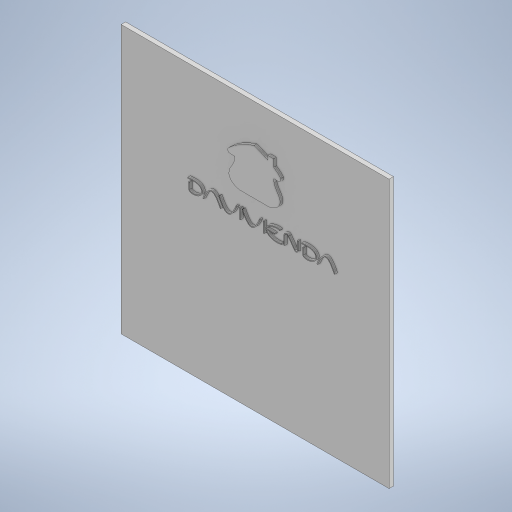
# Autodesk Inventor part: Davivienda
Saved by Autodesk Inventor 2023 (Build 270158000, 158)
## iProperties
Created: 2024-11-21
Part Number: Davivienda
Material: Generic
Document SubType Name: Modeling
Designer: Zenbook
Density: 1 g/cm^3
Appearance: Default
Author: Zenbook
Autodesk Inventor part; units mm, degrees
ref_plane "YZ Plane" through (0, 0, 0) normal (1, 0, 0) x (0, 1, 0)
ref_plane "XZ Plane" through (0, 0, 0) normal (0, 1, 0) x (-1, 0, 0)
ref_plane "XY Plane" through (0, 0, 0) normal (0, 0, 1) x (1, 0, 0)
sketch "Sketch2" plane through (0, 0, 0) normal (0, 0, 1) x (1, 0, 0)
  line L0 (0, 0) -> (300, 0)
  line L1 (300, 0) -> (300, 300)
  line L2 (300, 300) -> (0, 300)
  line L3 (0, 300) -> (0, 0)
  dimension "d0" = 300
  dimension "d1" = 300
  constraints: 8 end point, 2 parallel, 1 horizontal, 1 perpendicular
  measures "d0" distance of L2.end L1.end
  measures "d1" distance of L1.end L0.end
extrude "Extrusion1" add sketch "Sketch2" along normal blind 5
sketch "Sketch4" plane through (0, 0, 5) normal (0, 0, 1) x (1, 0, 0)
  line L0 (79.5564, 188.2855) -> (79.5564, 181.2855)
  line L1 (79.5564, 181.2855) -> (79.5564, 178.6599) construction
  line L2 (79.5564, 178.6599) -> (94.7024, 178.6599) construction
  line L3 (94.7024, 178.6599) -> (96.5971, 188.6652) construction
  line L4 (96.5971, 188.6652) -> (88.3362, 192.4913) construction
  line L5 (88.3362, 192.4913) -> (77.7258, 191.1271) construction
  spline S0 degree 4 poles (79.5564, 181.2855) (79.5564, 178.6599) (94.7024, 178.6599) (96.5971, 188.6652) (88.3362, 192.4913) (77.7258, 191.1271) knots 1 1 1 1 1 2 3 3 3 3 3
  line L6 (95.2867, 179.9727) -> (97.8294, 186.2811) construction
  line L7 (97.8294, 186.2811) -> (104.3309, 202.3418) construction
  line L8 (104.3309, 202.3418) -> (110.5428, 186.2811) construction
  line L9 (110.5428, 186.2811) -> (113.8579, 179.9727) construction
  spline S1 degree 4 poles (95.2867, 179.9727) (97.8294, 186.2811) (104.3309, 202.3418) (110.5428, 186.2811) (113.8579, 179.9727) knots 1 1 1 1 1 2 2 2 2 2
  line L10 (131.5825, 191.7075) -> (129.0398, 185.3991) construction
  line L11 (129.0398, 185.3991) -> (122.5383, 169.3383) construction
  line L12 (122.5383, 169.3383) -> (116.3264, 185.3991) construction
  line L13 (116.3264, 185.3991) -> (113.0113, 191.7075) construction
  spline S2 degree 4 poles (131.5825, 191.7075) (129.0398, 185.3991) (122.5383, 169.3383) (116.3264, 185.3991) (113.0113, 191.7075) knots 1 1 1 1 1 2 2 2 2 2
  spline S3 degree 4 poles (157.762, 191.8087) (155.2194, 185.5002) (148.7178, 169.4395) (142.5059, 185.5002) (139.1908, 191.8087) knots 1 1 1 1 1 2 2 2 2 2
  line L14 (157.762, 191.8087) -> (155.2194, 185.5002) construction
  line L15 (155.2194, 185.5002) -> (148.7178, 169.4395) construction
  line L16 (148.7178, 169.4395) -> (142.5059, 185.5002) construction
  line L17 (142.5059, 185.5002) -> (139.1908, 191.8087) construction
  line L18 (135.5149, 191.7075) -> (135.5149, 180.2075)
  line L19 (162.0018, 191.8085) -> (162.0018, 180.3085)
  line L20 (180.6346, 191.8085) -> (171.5415, 194.3115) construction
  line L21 (171.5415, 194.3115) -> (152.9228, 186.4259) construction
  line L22 (152.9228, 186.4259) -> (171.5415, 176.543) construction
  line L23 (171.5415, 176.543) -> (182.4118, 180.3085) construction
  spline S4 degree 4 poles (180.6346, 191.8085) (171.5415, 194.3115) (152.9228, 186.4259) (171.5415, 176.543) (182.4118, 180.3085) knots 1 1 1 1 1 2 2 2 2 2
  line L24 (165.8328, 186.4259) -> (174.8813, 186.4259)
  line L25 (186.057, 180.0241) -> (186.057, 189.935)
  line L26 (189.8603, 191.1584) -> (197.0204, 180.9967)
  line L27 (201.0713, 182.1524) -> (201.0713, 191.8085)
  arc A0 (189.8811, 191.1289) -> (186.057, 189.935) centre (188.1554, 189.935) ccw
  arc A1 (197.0204, 180.9967) -> (201.0713, 182.1524) centre (198.8441, 182.2817) ccw
  line L28 (207.2296, 188.507) -> (207.2296, 181.507)
  line L29 (207.2296, 181.507) -> (207.2296, 178.8814) construction
  line L30 (207.2296, 178.8814) -> (222.3756, 178.8814) construction
  line L31 (222.3756, 178.8814) -> (224.2703, 188.8868) construction
  line L32 (224.2703, 188.8868) -> (216.0093, 192.7129) construction
  line L33 (216.0093, 192.7129) -> (205.3989, 191.3487) construction
  spline S5 degree 4 poles (207.2296, 181.507) (207.2296, 178.8814) (222.3756, 178.8814) (224.2703, 188.8868) (216.0093, 192.7129) (205.3989, 191.3487) knots 1 1 1 1 1 2 3 3 3 3 3
  line L34 (222.9422, 180.0767) -> (225.4849, 186.3851) construction
  line L35 (225.4849, 186.3851) -> (231.9865, 202.4459) construction
  line L36 (231.9865, 202.4459) -> (238.1983, 186.3851) construction
  line L37 (238.1983, 186.3851) -> (241.5135, 180.0767) construction
  spline S6 degree 4 poles (222.9422, 180.0767) (225.4849, 186.3851) (231.9865, 202.4459) (238.1983, 186.3851) (241.5135, 180.0767) knots 1 1 1 1 1 2 2 2 2 2
  line L38 (135.9918, 208.9074) -> (168.4766, 208.9074)
  line L39 (167.2414, 253.646) -> (167.2414, 258.1826)
  line L40 (167.2414, 258.1826) -> (173.7908, 258.1826)
  line L41 (173.7908, 258.1826) -> (173.7908, 249.9244)
  line L42 (135.9918, 208.9074) -> (128.025, 210.0808) construction
  line L43 (128.025, 210.0808) -> (119.7557, 218.4745) construction
  line L44 (119.7557, 218.4745) -> (124.3195, 226.1379) construction
  line L45 (124.3195, 226.1379) -> (130.2483, 231.5726) construction
  line L46 (130.2483, 231.5726) -> (130.2483, 238.8487) construction
  spline S7 degree 4 poles (135.9918, 208.9074) (128.025, 210.0808) (119.7557, 218.4745) (124.3195, 226.1379) (130.2483, 231.5726) (130.2483, 238.8487) knots 1 1 1 1 1 2 3 3 3 3 3
  line L47 (168.4766, 208.9074) -> (175.8602, 210.0808) construction
  line L48 (175.8602, 210.0808) -> (186.1394, 218.4745) construction
  line L49 (186.1394, 218.4745) -> (179.0921, 227.5218) construction
  line L50 (179.0921, 227.5218) -> (173.9355, 231.5726) construction
  line L51 (173.9355, 231.5726) -> (173.9355, 238.8487) construction
  spline S8 degree 4 poles (168.4766, 208.9074) (175.8602, 210.0808) (186.1394, 218.4745) (179.0921, 227.5218) (173.9355, 231.5726) (173.9355, 238.8487) knots 1 1 1 1 1 2 3 3 3 3 3
  line L52 (123.2696, 243.6155) -> (134.5896, 254.6512) construction
  line L53 (134.5896, 254.6512) -> (152.0248, 260.2524) construction
  spline S9 degree 2 poles (123.2696, 243.6155) (134.5896, 254.6512) (152.0248, 260.2524) knots 1 1 1 2 2 2
  line L54 (152.0248, 260.2524) -> (160.8389, 256.9124) construction
  line L55 (179.2014, 246.4492) -> (181.8101, 243.0596) construction
  arc A2 (123.2696, 243.6155) -> (124.9575, 238.8487) centre (124.9575, 241.5309) ccw
  arc A3 (179.0921, 238.8487) -> (181.8101, 243.0596) centre (179.0921, 241.8313) ccw
  line L56 (124.9575, 238.8487) -> (130.2483, 238.8487)
  line L57 (173.9355, 238.8487) -> (179.0921, 238.8487)
  spline S10 degree 2 poles (152.0248, 260.2524) (160.8389, 256.9124) (167.2414, 253.646) knots 0 0 0 1 1 1
  spline S11 degree 2 poles (173.7908, 249.9244) (179.2014, 246.4492) (181.8101, 243.0596) knots 0 0 0 1 1 1
  line L58 (160.8389, 256.9124) -> (167.2414, 253.646) construction
  line L59 (173.7908, 249.9244) -> (179.2014, 246.4492) construction
  point P0 (0, 0)
  point P1 (175.3935, 251.397)
  dimension "d11" = 7
  dimension "d28" = 11.5
  dimension "d29" = 11.5
  dimension "d42" = 7
  constraints: 28 end point, 9 point on circle, 7 vertical, 6 tangent, 4 centre point, 4 horizontal, 4 perpendicular, 1 point on line, 37 other
  measures "d11" distance of L0.start L0.end
  measures "d28" distance of L18.start L18.end
  measures "d29" distance of L19.start L19.end
  measures "d42" distance of L28.start L29.start
extrude "Extrusion2" add sketch "Sketch4" along normal blind 3
sketch "Sketch6" plane through (0, 0, 5) normal (0, 0, 1) x (1, 0, 0)
  line L0 (79.5564, 188.2855) -> (79.5564, 181.2855)
  line L1 (79.5564, 181.2855) -> (79.5564, 178.6599) construction
  line L2 (79.5564, 178.6599) -> (94.7024, 178.6599) construction
  line L3 (94.7024, 178.6599) -> (96.5971, 188.6652) construction
  line L4 (96.5971, 188.6652) -> (88.3362, 192.4913) construction
  line L5 (88.3362, 192.4913) -> (77.7258, 191.1271) construction
  spline S0 degree 4 poles (79.5564, 181.2855) (79.5564, 178.6599) (94.7024, 178.6599) (96.5971, 188.6652) (88.3362, 192.4913) (77.7258, 191.1271) knots 1 1 1 1 1 2 3 3 3 3 3
  line L6 (95.2867, 179.9727) -> (97.8294, 186.2811) construction
  line L7 (97.8294, 186.2811) -> (104.3309, 202.3418) construction
  line L8 (104.3309, 202.3418) -> (110.5428, 186.2811) construction
  line L9 (110.5428, 186.2811) -> (113.8579, 179.9727) construction
  spline S1 degree 4 poles (95.2867, 179.9727) (97.8294, 186.2811) (104.3309, 202.3418) (110.5428, 186.2811) (113.8579, 179.9727) knots 1 1 1 1 1 2 2 2 2 2
  spline S2 degree 4 poles (131.5825, 191.7075) (129.0398, 185.3991) (122.5383, 169.3383) (116.3264, 185.3991) (113.0113, 191.7075) knots 1 1 1 1 1 2 2 2 2 2
  line L10 (131.5825, 191.7075) -> (129.0398, 185.3991) construction
  line L11 (129.0398, 185.3991) -> (122.5383, 169.3383) construction
  line L12 (122.5383, 169.3383) -> (116.3264, 185.3991) construction
  line L13 (116.3264, 185.3991) -> (113.0113, 191.7075) construction
  spline S3 degree 4 poles (157.762, 191.8087) (155.2194, 185.5002) (148.7178, 169.4395) (142.5059, 185.5002) (139.1908, 191.8087) knots 1 1 1 1 1 2 2 2 2 2
  line L14 (157.762, 191.8087) -> (155.2194, 185.5002) construction
  line L15 (155.2194, 185.5002) -> (148.7178, 169.4395) construction
  line L16 (148.7178, 169.4395) -> (142.5059, 185.5002) construction
  line L17 (142.5059, 185.5002) -> (139.1908, 191.8087) construction
  line L18 (135.5149, 191.7075) -> (135.5149, 180.2075)
  line L19 (162.0018, 191.8085) -> (162.0018, 180.3085)
  line L20 (180.6346, 191.8085) -> (171.5415, 194.3115) construction
  line L21 (171.5415, 194.3115) -> (152.9228, 186.4259) construction
  line L22 (152.9228, 186.4259) -> (171.5415, 176.543) construction
  line L23 (171.5415, 176.543) -> (182.4118, 180.3085) construction
  spline S4 degree 4 poles (180.6346, 191.8085) (171.5415, 194.3115) (152.9228, 186.4259) (171.5415, 176.543) (182.4118, 180.3085) knots 1 1 1 1 1 2 2 2 2 2
  line L24 (165.8328, 186.4259) -> (174.8813, 186.4259)
  line L25 (186.057, 180.0241) -> (186.057, 189.935)
  line L26 (189.8603, 191.1584) -> (197.0204, 180.9967)
  line L27 (201.0713, 182.1524) -> (201.0713, 191.8085)
  arc A0 (189.8811, 191.1289) -> (186.057, 189.935) centre (188.1554, 189.935) ccw
  arc A1 (197.0204, 180.9967) -> (201.0713, 182.1524) centre (198.8441, 182.2817) ccw
  spline S5 degree 4 poles (207.2296, 181.507) (207.2296, 178.8814) (222.3756, 178.8814) (224.2703, 188.8868) (216.0093, 192.7129) (205.3989, 191.3487) knots 1 1 1 1 1 2 3 3 3 3 3
  line L28 (207.2296, 181.507) -> (207.2296, 178.8814) construction
  line L29 (207.2296, 178.8814) -> (222.3756, 178.8814) construction
  line L30 (222.3756, 178.8814) -> (224.2703, 188.8868) construction
  line L31 (224.2703, 188.8868) -> (216.0093, 192.7129) construction
  line L32 (216.0093, 192.7129) -> (205.3989, 191.3487) construction
  line L33 (207.2296, 188.507) -> (207.2296, 181.507)
  spline S6 degree 4 poles (222.9422, 180.0767) (225.4849, 186.3851) (231.9865, 202.4459) (238.1983, 186.3851) (241.5135, 180.0767) knots 1 1 1 1 1 2 2 2 2 2
  line L34 (222.9422, 180.0767) -> (225.4849, 186.3851) construction
  line L35 (225.4849, 186.3851) -> (231.9865, 202.4459) construction
  line L36 (231.9865, 202.4459) -> (238.1983, 186.3851) construction
  line L37 (238.1983, 186.3851) -> (241.5135, 180.0767) construction
  line L38 (78.5564, 181.2855) -> (78.5564, 188.2855)
  line L39 (136.5149, 191.7075) -> (136.5149, 180.2075)
  line L40 (163.0018, 191.8085) -> (163.0018, 180.3085)
  line L41 (165.8565, 185.4259) -> (174.8813, 185.4259)
  line L42 (185.057, 180.0241) -> (185.057, 189.935)
  arc A2 (190.7035, 191.6979) -> (185.057, 189.935) centre (188.1554, 189.935) ccw
  line L43 (190.6778, 191.7344) -> (197.8379, 181.5727)
  arc A3 (197.8379, 181.5727) -> (200.0713, 182.1857) centre (198.8441, 182.2817) ccw
  line L44 (200.0713, 182.1857) -> (200.0713, 191.8085)
  line L45 (206.2296, 181.507) -> (206.2296, 188.507)
  line L46 (79.5564, 188.2855) -> (78.5564, 188.2855)
  line L47 (77.7258, 191.1271) -> (77.5982, 192.1189)
  line L48 (95.2867, 179.9727) -> (94.3592, 180.3465)
  line L49 (113.8579, 179.9727) -> (114.7431, 180.4378)
  line L50 (112.1261, 191.2423) -> (113.0113, 191.7075)
  line L51 (132.51, 191.3337) -> (131.5825, 191.7075)
  line L52 (135.5149, 191.7075) -> (136.5149, 191.7075)
  line L53 (135.5149, 180.2075) -> (136.5149, 180.2075)
  line L54 (138.3056, 191.3435) -> (139.1908, 191.8087)
  line L55 (157.762, 191.8087) -> (158.6895, 191.4348)
  line L56 (162.0018, 191.8085) -> (163.0018, 191.8085)
  line L57 (162.0018, 180.3085) -> (163.0018, 180.3085)
  line L58 (182.7391, 179.3635) -> (182.4118, 180.3085)
  line L59 (174.8813, 185.4259) -> (174.8813, 186.4259)
  line L60 (185.057, 180.0241) -> (186.057, 180.0241)
  line L61 (200.0713, 191.8085) -> (201.0713, 191.8085)
  line L62 (205.3989, 191.3487) -> (205.2714, 192.3405)
  line L63 (206.2296, 188.507) -> (207.2296, 188.507)
  line L64 (222.0147, 180.4505) -> (222.9422, 180.0767)
  line L65 (241.5135, 180.0767) -> (242.3987, 180.5419)
  line L66 (180.6346, 191.8085) -> (180.9, 192.7726)
  spline S7 degree 5 poles (77.5982, 192.1189) (78.6162, 192.2498) (79.6368, 192.3603) (80.6599, 192.4464) (82.4837, 192.5473) (84.3098, 192.5266) (85.1087, 192.4899) (86.5329, 192.3645) (87.9377, 192.1029) (88.5503, 191.9568) (89.6455, 191.6249) (90.6851, 191.1491) (91.1369, 190.903) (91.9401, 190.3755) (92.6391, 189.7178) (92.9357, 189.3838) (93.4406, 188.6884) (93.8, 187.9087) (93.9352, 187.5178) (94.1241, 186.7215) (94.155, 185.9038) (94.1312, 185.4984) (94.0058, 184.6818) (93.7337, 183.9014) (93.5597, 183.5177) (93.1316, 182.7565) (92.5837, 182.0758) (92.2726, 181.7464) (91.5774, 181.1067) (90.8033, 180.5642) (90.3835, 180.3067) (89.4876, 179.8223) (88.5464, 179.433) (88.0508, 179.2556) (87.0359, 178.9432) (85.9973, 178.7219) (85.4688, 178.633) (84.4327, 178.5055) (83.3893, 178.4743) (82.8811, 178.4845) (81.9175, 178.556) (80.9731, 178.7614) (80.5348, 178.8931) (79.6638, 179.2662) (78.9659, 179.9065) (78.6841, 180.3256) (78.5566, 180.8089) (78.5564, 181.2855) knots 0 0 0 0 0 0 0.12687 0.12687 0.12687 0.225646 0.225646 0.225646 0.30335 0.30335 0.30335 0.36672 0.36672 0.36672 0.421609 0.421609 0.421609 0.472388 0.472388 0.472388 0.522285 0.522285 0.522285 0.5741 0.5741 0.5741 0.629898 0.629898 0.629898 0.690657 0.690657 0.690657 0.755632 0.755632 0.755632 0.821798 0.821798 0.821798 0.884532 0.884532 0.884532 0.940955 0.940955 0.940955 1 1 1 1 1 1
  spline S8 degree 5 poles (94.3592, 180.3465) (94.6691, 181.116) (94.9805, 181.8849) (95.3032, 182.6493) (96.0129, 184.2544) (96.7976, 185.8242) (97.2377, 186.6387) (98.1315, 188.1503) (99.1811, 189.559) (99.7178, 190.1922) (100.829, 191.292) (102.1665, 192.0911) (102.8464, 192.374) (104.2911, 192.6572) (105.7357, 192.373) (106.4176, 192.0904) (107.7678, 191.2937) (108.8988, 190.2004) (109.4502, 189.57) (110.5378, 188.1657) (111.4812, 186.6617) (111.9519, 185.8509) (112.8049, 184.2881) (113.6061, 182.6979) (113.9804, 181.9424) (114.3511, 181.1846) (114.7431, 180.4378) knots 0 0 0 0 0 0 0.124856 0.124856 0.124856 0.264073 0.264073 0.264073 0.388815 0.388815 0.388815 0.497298 0.497298 0.497298 0.606144 0.606144 0.606144 0.732055 0.732055 0.732055 0.87307 0.87307 0.87307 1 1 1 1 1 1
  spline S9 degree 5 poles (132.51, 191.3337) (132.2, 190.5642) (131.8887, 189.7952) (131.566, 189.0309) (130.8563, 187.4257) (130.0715, 185.8559) (129.6315, 185.0414) (128.7377, 183.5299) (127.6881, 182.1212) (127.1514, 181.488) (126.0402, 180.3882) (124.7026, 179.5891) (124.0227, 179.3061) (122.5781, 179.023) (121.1335, 179.3071) (120.4516, 179.5897) (119.1014, 180.3864) (117.9703, 181.4798) (117.4189, 182.1102) (116.3314, 183.5145) (115.388, 185.0184) (114.9173, 185.8293) (114.0642, 187.392) (113.2631, 188.9823) (112.8887, 189.7378) (112.518, 190.4956) (112.1261, 191.2423) knots 0 0 0 0 0 0 0.124856 0.124856 0.124856 0.264073 0.264073 0.264073 0.388815 0.388815 0.388815 0.497298 0.497298 0.497298 0.606144 0.606144 0.606144 0.732055 0.732055 0.732055 0.87307 0.87307 0.87307 1 1 1 1 1 1
  spline S10 degree 5 poles (158.6895, 191.4348) (158.3796, 190.6653) (158.0682, 189.8964) (157.7455, 189.1321) (157.0358, 187.5269) (156.2511, 185.9571) (155.811, 185.1426) (154.9172, 183.631) (153.8676, 182.2223) (153.3309, 181.5891) (152.2197, 180.4894) (150.8822, 179.6902) (150.2023, 179.4073) (148.7576, 179.1242) (147.3131, 179.4083) (146.6311, 179.6909) (145.2809, 180.4876) (144.1499, 181.5809) (143.5985, 182.2113) (142.5109, 183.6156) (141.5675, 185.1196) (141.0968, 185.9304) (140.2438, 187.4932) (139.4426, 189.0834) (139.0683, 189.8389) (138.6976, 190.5967) (138.3056, 191.3435) knots 0 0 0 0 0 0 0.124856 0.124856 0.124856 0.264073 0.264073 0.264073 0.388815 0.388815 0.388815 0.497298 0.497298 0.497298 0.606144 0.606144 0.606144 0.732055 0.732055 0.732055 0.87307 0.87307 0.87307 1 1 1 1 1 1
  spline S11 degree 5 poles (180.9, 192.7726) (179.961, 193.031) (178.9925, 193.1803) (178.0185, 193.2514) (176.0567, 193.2587) (174.1104, 193.0159) (173.1409, 192.8357) (171.3349, 192.3844) (169.6037, 191.6996) (168.8139, 191.3211) (167.4152, 190.5034) (166.2218, 189.4139) (165.7328, 188.8525) (164.9739, 187.6153) (164.7208, 186.1884) (164.7518, 185.476) (165.1202, 184.0479) (165.9664, 182.8345) (166.4989, 182.2761) (167.7984, 181.1743) (169.2947, 180.3514) (170.1475, 179.9675) (172.0371, 179.2718) (174.0038, 178.8379) (175.0707, 178.6746) (177.2645, 178.4828) (179.4643, 178.6019) (180.5798, 178.7493) (181.6801, 178.9966) (182.7391, 179.3635) knots 0 0 0 0 0 0 0.11949 0.11949 0.11949 0.240188 0.240188 0.240188 0.347394 0.347394 0.347394 0.437627 0.437627 0.437627 0.522195 0.522195 0.522195 0.615974 0.615974 0.615974 0.730426 0.730426 0.730426 0.862485 0.862485 0.862485 1 1 1 1 1 1
  spline S12 degree 5 poles (205.2714, 192.3405) (206.2894, 192.4714) (207.3099, 192.5819) (208.333, 192.668) (210.1569, 192.7689) (211.983, 192.7482) (212.7819, 192.7115) (214.206, 192.5861) (215.6109, 192.3244) (216.2234, 192.1784) (217.3186, 191.8464) (218.3583, 191.3707) (218.8101, 191.1245) (219.6132, 190.597) (220.3122, 189.9393) (220.6089, 189.6054) (221.1138, 188.91) (221.4732, 188.1302) (221.6084, 187.7394) (221.7973, 186.9431) (221.8282, 186.1254) (221.8043, 185.7199) (221.679, 184.9033) (221.4069, 184.123) (221.2328, 183.7393) (220.8047, 182.978) (220.2569, 182.2974) (219.9458, 181.968) (219.2505, 181.3283) (218.4765, 180.7858) (218.0566, 180.5283) (217.1608, 180.0439) (216.2195, 179.6546) (215.724, 179.4772) (214.709, 179.1648) (213.6704, 178.9435) (213.1419, 178.8546) (212.1058, 178.7271) (211.0625, 178.6959) (210.5542, 178.7061) (209.5906, 178.7776) (208.6462, 178.983) (208.2079, 179.1147) (207.337, 179.4878) (206.6391, 180.128) (206.3572, 180.5472) (206.2297, 181.0305) (206.2296, 181.507) knots 0 0 0 0 0 0 0.12687 0.12687 0.12687 0.225646 0.225646 0.225646 0.30335 0.30335 0.30335 0.36672 0.36672 0.36672 0.421609 0.421609 0.421609 0.472388 0.472388 0.472388 0.522285 0.522285 0.522285 0.5741 0.5741 0.5741 0.629898 0.629898 0.629898 0.690657 0.690657 0.690657 0.755632 0.755632 0.755632 0.821798 0.821798 0.821798 0.884532 0.884532 0.884532 0.940955 0.940955 0.940955 1 1 1 1 1 1
  spline S13 degree 5 poles (222.0147, 180.4505) (222.3247, 181.22) (222.6361, 181.989) (222.9587, 182.7533) (223.6685, 184.3585) (224.4532, 185.9283) (224.8933, 186.7428) (225.787, 188.2543) (226.8367, 189.663) (227.3734, 190.2962) (228.4846, 191.396) (229.8221, 192.1951) (230.502, 192.4781) (231.9466, 192.7612) (233.3912, 192.4771) (234.0732, 192.1945) (235.4234, 191.3978) (236.5544, 190.3044) (237.1058, 189.674) (238.1934, 188.2697) (239.1368, 186.7658) (239.6075, 185.9549) (240.4605, 184.3922) (241.2617, 182.8019) (241.636, 182.0464) (242.0067, 181.2886) (242.3987, 180.5419) knots 0 0 0 0 0 0 0.124856 0.124856 0.124856 0.264073 0.264073 0.264073 0.388815 0.388815 0.388815 0.497298 0.497298 0.497298 0.606144 0.606144 0.606144 0.732055 0.732055 0.732055 0.87307 0.87307 0.87307 1 1 1 1 1 1
  point P0 (0, 0)
  point P1 (190.7008, 191.7018)
  dimension "d75" = 1
  dimension "d76" = 1
  dimension "d77" = 1
  dimension "d79" = 1
  dimension "d81" = 1
  dimension "d85" = 1
  dimension "d86" = 1
  dimension "d71" = 7
  dimension "d72" = 11.5
  dimension "d73" = 11.5
  dimension "d74" = 7
  dimension "d78" = 1
  dimension "d80" = 1
  dimension "d82" = 1
  dimension "d83" = 1
  dimension "d84" = 1
  constraints: 74 end point, 14 parallel, 9 point on circle, 6 perpendicular, 6 vertical, 4 centre point, 2 tangent, 1 horizontal, 1 point on line, 47 other
  measures "d71" distance of L0.start L0.end
  measures "d72" distance of L18.start L18.end
  measures "d73" distance of L19.start L19.end
  measures "d74" distance of L33.start L33.end
  measures "d78" distance between parallel lines of L18 L39
  measures "d80" distance between parallel lines of L19 L40
  measures "d82" distance between parallel lines of L24 L41
  measures "d83" distance between parallel lines of L25 L42
  measures "d84" distance between parallel lines of L26 L43
extrude "Extrusion3" add sketch "Sketch6" along normal blind 3
body "Solid1"
